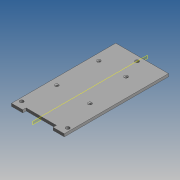
# Autodesk Inventor part: P042_BoitierCouvercleV4_moduleHaut
Saved by Autodesk Inventor 2021.3 (Build 253353000, 353)
## iProperties
Created: 2021-12-17
Part Number: P042_BoitierCouvercleV4_moduleHaut
Material: Générique
Document SubType Name: Modeling
Designer: gabri
Density: 1 g/cm^3
Appearance: Par défaut
Author: gabri
Autodesk Inventor part; units mm, degrees
ref_plane "XZ Plane" through (0, 0, 0) normal (0, 1, 0) x (-1, 0, 0)
ref_plane "XY Plane" through (0, 0, 0) normal (0, 0, 1) x (1, 0, 0)
sketch "Sketch2" plane through (0, 0, 0) normal (0, 0, 1) x (1, 0, 0)
  line L0 (39.25, -77.5) -> (-39.25, -77.5)
  line L1 (-39.25, -77.5) -> (-39.25, 77.5)
  line L2 (-39.25, 77.5) -> (39.25, 77.5)
  line L3 (39.25, 77.5) -> (39.25, -77.5)
  line L4 (39.25, -77.5) -> (-39.25, 77.5) construction
  line L5 (-39.25, -77.5) -> (39.25, 77.5) construction
  point P0 (0, 0)
  dimension "d0" = 78.5
  dimension "d1" = 155
  constraints: 12 end point, 2 midpoint, 2 parallel, 1 horizontal, 1 perpendicular
  measures "d0" distance of L1.end L2.end
  measures "d1" distance between parallel lines of L0 L2
extrude "Extrusion1" add sketch "Sketch2" along normal blind 4
sketch "Sketch3" plane through (0, 0, 4) normal (0, 0, 1) x (1, 0, 0)
  line L0 (0, 108.5) -> (0, -108.5) construction
  line L1 (39.25, 77.5) -> (-39.25, 77.5) construction
  point P0 (0, 0)
  point P1 (0, 70)
  point P2 (-34.25, -67.5)
  point P3 (34.25, -67.5)
  dimension "d4" = 34.25
  dimension "d5" = 34.25
  dimension "d6" = 137.5
  dimension "d8" = 7.5
  dimension "d9" = 137.5
  constraints: 1 point on line
  measures "d4" distance from line of L0 point (-34.25, -67.5)
  measures "d5" distance from line of L0 point (34.25, -67.5)
  measures "d6" vertical distance of point (0, 70) point (-34.25, -67.5)
  measures "d8" distance from line of L1 point (0, 70)
  measures "d9" vertical distance of point (0, 70) point (34.25, -67.5)
hole "Hole1" at (0, 70, 4) at (-34.25, -67.5, 4) at (34.25, -67.5, 4) direction (0, 0, -1) diameter 5.5 depth 9.5
sketch "Sketch4" plane through (0, 0, 0) normal (0, 0, -1) x (-1, 0, 0)
  line L0 (-27.565, 44.5) -> (-27.565, 40.5) construction
  line L1 (-27.565, 40.5) -> (-37.565, 40.5) construction
  line L2 (-37.565, 40.5) -> (-37.565, 32.5) construction
  line L3 (-37.565, 32.5) -> (-27.565, 32.5) construction
  line L4 (-27.565, 32.5) -> (-27.565, -48.52) construction
  line L5 (-27.565, -48.52) -> (-10.565, -48.52) construction
  line L6 (-10.565, -48.52) -> (-10.565, -58.52) construction
  line L7 (-10.565, -58.52) -> (-2.565, -58.52) construction
  line L8 (-2.565, -58.52) -> (-2.565, -48.52) construction
  line L9 (-2.565, -48.52) -> (37.5, -48.52) construction
  line L10 (37.5, -48.52) -> (37.5, 44.5) construction
  line L11 (37.5, 44.5) -> (28.5, 44.5) construction
  line L12 (28.5, 44.5) -> (26.5, 46.5) construction
  line L13 (26.5, 46.5) -> (18.5, 46.5) construction
  line L14 (18.5, 46.5) -> (18.5, 56.5) construction
  line L15 (18.5, 56.5) -> (7.5, 56.5) construction
  line L16 (7.5, 56.5) -> (7.5, 46.5) construction
  line L17 (7.5, 46.5) -> (-6.565, 46.5) construction
  line L18 (-6.565, 46.5) -> (-8.565, 44.5) construction
  line L19 (-8.565, 44.5) -> (-27.565, 44.5) construction
  circle A0 centre (29.081, 42.025) radius 1.6 construction
  circle A1 centre (-11.625, 42.025) radius 1.6 construction
  circle A2 centre (28.95, -20.606) radius 1.6 construction
  circle A3 centre (-19.179, -19.336) radius 1.6 construction
  point P0 (0, 0)
  constraints: 4 coincident
hole "Hole2" at (-29.081, 42.025, 0) at (-28.95, -20.606, 0) at (19.179, -19.336, 0) at (11.625, 42.025, 0) direction (0, 0, 1) diameter 3.5 depth 9.5
chamfer "Chamfer1" distance 1 angle 45 4 edges at (11.625, 40.275, 4) (19.179, -21.086, 4) (-28.95, -22.356, 4) (-29.081, 40.275, 4)
sketch "Sketch6" plane through (0, 0, 4) normal (0, 0, 1) x (1, 0, 0)
  circle A0 centre (-28.95, -20.606) radius 2.75 construction
  circle A1 centre (11.625, 42.025) radius 2.75 construction
  circle A2 centre (-34.25, -67.5) radius 2.75 construction
  circle A3 centre (0, 70) radius 2.75 construction
  circle A4 centre (34.25, -67.5) radius 2.75 construction
  line L0 (39.25, 77.5) -> (-39.25, 77.5) construction
  line L1 (-39.25, 77.5) -> (-39.25, -77.5) construction
  line L2 (-39.25, -77.5) -> (39.25, -77.5) construction
  line L3 (39.25, -77.5) -> (39.25, 77.5) construction
  circle A5 centre (19.179, -19.336) radius 2.75 construction
  circle A6 centre (-29.081, 42.025) radius 2.75 construction
  line L4 (22.5, -72.5) -> (-22.5, -72.5)
  line L5 (-22.5, -72.5) -> (-22.5, -77.5)
  line L6 (-22.5, -77.5) -> (22.5, -77.5)
  line L7 (22.5, -77.5) -> (22.5, -72.5)
  line L8 (0, 108.5) -> (0, -108.5) construction
  point P0 (0, 0)
  dimension "d33" = 45
  dimension "d34" = 5
  dimension "d35" = 22.5
  constraints: 8 end point, 2 parallel, 1 horizontal, 1 perpendicular, 1 point on line
  measures "d33" distance of L4.start L4.end
  measures "d34" distance of L4.end L5.end
  measures "d35" distance between parallel lines of L8 L7
extrude "Extrusion3" cut sketch "Sketch6" against normal blind 10
equation "\"d35\" = 0.5 * d33"
body "Solid1"
